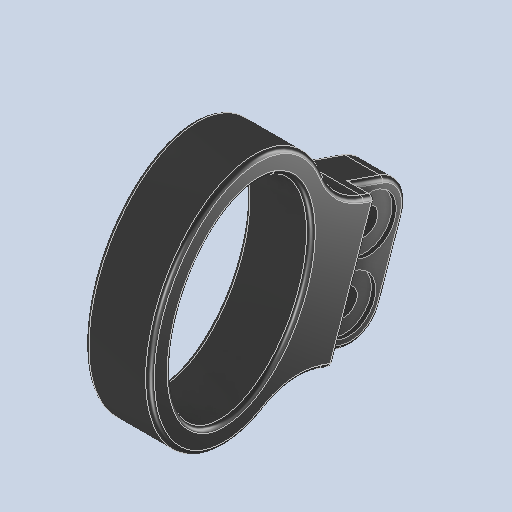
# Autodesk Inventor part: TorsoFrontBumper
Saved by Autodesk Inventor 2024.2 (Build 282272000, 272)
## iProperties
Created: 2024-01-21
Part Number: TorsoFrontBumper
Material: ABS Plastic
Document SubType Name: Modeling
Designer: Masato Kubotera
Density: 1.06 g/cm^3
Appearance: Glossy - Black
Mass: 18.7145 g
Surface Area: 72.9359 cm^2
Volume: 17.6552 cm^3
Catalog Web Link: https://www.poly-maker.jp/polyflex-tpu90.html
Author: Masato Kubotera
Autodesk Inventor part; units mm, degrees
ref_plane "YZ Plane" through (0, 0, 0) normal (1, 0, 0) x (0, 1, 0)
ref_plane "XZ Plane" through (0, 0, 0) normal (0, 1, 0) x (-1, 0, 0)
ref_plane "XY Plane" through (0, 0, 0) normal (0, 0, 1) x (1, 0, 0)
derived "TorsoSideFrame.ipt"
sketch "Sketch5" plane through (0, 0, 0) normal (0, 1, 0) x (-1, 0, 0)
  ellipse E0 centre (-84.0749, 16.6972) end of major axis (-76.7401, 37.9681) minor radius 15 projected
  ellipse E1 centre (-84.0749, 16.6972) end of major axis (-93.0397, -9.3006) minor radius 20 projected
  line L0 (-63.4041, 25.9649) -> (-39.2683, 17.6422) projected
  line L1 (-49.374, -11.6643) -> (-73.5098, -3.3416) projected
  line L2 (-39.2683, 17.6422) -> (-49.374, -11.6643) projected
  line L3 (-48.2759, 36) -> (-65, -12.5) projected
  point P0 (0, 0)
  point P1 (-54.4839, -1.1756)
  point P2 (-49.757, 12.5323)
  point P3 (-63.0819, -6.9375)
  point P4 (-52.9762, 22.3691)
  constraints: 1 other
extrude "Extrusion2" add sketch "Sketch5" against normal blind 10
extrude "Extrusion5" add sketch "Sketch5" along normal blind 5 contours E1 | E1 L0 L3 L1
hole "Hole3" at (54.4839, 0, -1.1756) at (49.757, 0, 12.5323) direction (0, -1, 0) diameter 6 end through all counterbore diameter 12.5 counterbore depth 1
fillet "Fillet9" radius 15 4 edges at (63.4041, -5, 25.9649) (63.4041, 2.5, 25.9649) (73.5098, -5, -3.3416) (73.5098, 2.5, -3.3416)
fillet "Fillet10" radius 1 17 edges at (91.4097, -10, -4.5737) (102.9824, -10, 23.217) (91.4097, 5, -4.5737) (44.3211, -10, 2.989) (57.6584, -10, -8.8076) (47.5527, -10, 20.4989) (52.9762, 2.5, 22.3691) (63.0819, 2.5, -6.9375) (46.1222, 0, 20.0057) (56.2279, 0, -9.3009) (44.3211, 0, 2.989) (54.4066, 5, 22.8624) (102.9824, 5, 23.217) (72.3744, 5, -5.211) (64.5123, 5, -6.4442) (61.3578, 5, 26.7371) (58.029, 5, 7.7158)
fillet "Fillet11" radius 7.5 2 edges at (39.2683, -5, 17.6422) (49.374, -5, -11.6643)
sketch "Sketch1" plane through (0, 0, 0) normal (0, 1, 0) x (-1, 0, 0)
  circle A0 centre (0, 0) radius 18.75 projected
  line L0 (0, 0) -> (0, -161.5) projected
  circle A1 centre (0, 0) radius 29 construction
  line L1 (0, 0) -> (0, 36) projected
  line L2 (0, 36) -> (-48.2759, 36) projected
  line L3 (-65, -12.5) -> (-65, -118) projected
  line L4 (-50, -161.5) -> (-35, -161.5) projected
  line L5 (-35, -161.5) -> (-35, -166.5) projected
  line L6 (-35, -166.5) -> (-10, -166.5) projected
  line L7 (-10, -166.5) -> (-10, -161.5) projected
  line L8 (-10, -161.5) -> (0, -161.5) projected
  line L9 (-60, -40.225) -> (-65, -40.225) projected
  line L10 (-44, -161.5) -> (-44, -155.5) construction
  line L11 (-22.5, -166.5) -> (-22.5, -161.5) construction
  arc A2 (-6, -161.5) -> (-10, -161.5) centre (-8, -161.5) ccw projected
  arc A3 (-35, -161.5) -> (-39, -161.5) centre (-37, -161.5) ccw projected
  line L12 (-65, -12.5) -> (-60, -12.5) construction
  line L13 (-60, -12.5) -> (-60, -106) construction
  line L14 (-62.5, -12.5) -> (-62.5, -106) construction
  line L15 (-65, -40.25) -> (-60, -40.25) construction
  arc A4 (-60, -44.225) -> (-60, -40.225) centre (-60, -42.225) ccw projected
  line L16 (-60, -111) -> (0, -111) construction
  line L17 (-60, -106) -> (0, -106) construction
  line L18 (-60, -108.5) -> (-17.75, -108.5) construction
  line L19 (-9.95, -111.05) -> (-25.55, -111.05) projected
  line L20 (-25.55, -111.05) -> (-25.55, -105.95) projected
  line L21 (-25.55, -105.95) -> (-9.95, -105.95) projected
  line L22 (-9.95, -105.95) -> (-9.95, -111.05) projected
  line L23 (-9.95, -111.05) -> (-25.55, -105.95) construction
  line L24 (-25.55, -111.05) -> (-9.95, -105.95) construction
  line L25 (-25.5, -106) -> (-25.5, -111) construction
  arc A5 (-21.55, -105.95) -> (-25.55, -105.95) centre (-23.55, -105.95) ccw projected
  arc A6 (-25.55, -111.05) -> (-21.55, -111.05) centre (-23.55, -111.05) ccw projected
  line L26 (-22.5, -76.5) -> (-42.5, -76.5) construction
  line L27 (-42.5, -76.5) -> (-42.5, -96.5) construction
  line L28 (-42.5, -96.5) -> (-22.5, -96.5) construction
  line L29 (-22.5, -96.5) -> (-22.5, -76.5) construction
  line L30 (-22.5, -76.5) -> (-42.5, -96.5) construction
  line L31 (-42.5, -76.5) -> (-22.5, -96.5) construction
  line L32 (-45, -74) -> (-20, -74) construction
  line L33 (-20, -74) -> (-20, -99) construction
  line L34 (-20, -99) -> (-45, -99) construction
  line L35 (-45, -99) -> (-45, -74) construction
  line L36 (-45, -74) -> (-20, -99) construction
  line L37 (-20, -74) -> (-45, -99) construction
  line L38 (-50, 31) -> (0, 31) construction
  line L39 (-38.05, 31.05) -> (-13.95, 31.05) projected
  line L40 (-13.95, 31.05) -> (-13.95, 25.95) projected
  line L41 (-13.95, 25.95) -> (-38.05, 25.95) projected
  line L42 (-38.05, 25.95) -> (-38.05, 31.05) projected
  line L43 (-38.05, 31.05) -> (-13.95, 25.95) construction
  line L44 (-13.95, 31.05) -> (-38.05, 25.95) construction
  line L45 (-38.05, 28.5) -> (-13.95, 28.5) construction
  line L46 (-38, 31) -> (-38, 26) construction
  line L47 (-26, 31.05) -> (-26, 25.95) construction
  line L48 (-14, 31) -> (-14, 26) construction
  arc A7 (-34.05, 31.05) -> (-38.05, 31.05) centre (-36.05, 31.05) ccw projected
  arc A8 (-38.05, 25.95) -> (-34.05, 25.95) centre (-36.05, 25.95) ccw projected
  arc A9 (-13.95, 31.05) -> (-17.95, 31.05) centre (-15.95, 31.05) ccw projected
  arc A10 (-17.95, 25.95) -> (-13.95, 25.95) centre (-15.95, 25.95) ccw projected
  line L49 (-46.0671, -156.5) -> (-3.5, -156.5) projected
  arc A11 (-47.9578, -155.152) -> (-46.0671, -156.5) centre (-46.0671, -154.5) ccw projected
  arc A12 (-3.5, -156.5) -> (-1.5, -154.5) centre (-3.5, -154.5) ccw projected
  line L50 (-56, -105.25) -> (-29.4627, -105.25) projected
  circle A13 centre (-41.25, -65.25) radius 2 construction
  line L51 (-1.5, -63.25) -> (-56, -63.25) projected
  line L52 (0, 0) -> (-29, 0) construction
  line L53 (-60, -111.75) -> (-29.4627, -111.75) projected
  arc A14 (-27.6434, -112.9192) -> (-20.2699, -114.1308) centre (-23.55, -111.05) ccw projected
  line L54 (-1.5, -154.5) -> (-1.5, -113.75) projected
  arc A15 (-1.5, -113.75) -> (-3.5, -111.75) centre (-3.5, -113.75) ccw projected
  arc A16 (-27.6434, -112.9192) -> (-29.4627, -111.75) centre (-29.4627, -113.75) ccw projected
  circle A17 centre (-33.5, -108.5) radius 1.75 construction
  arc A18 (-18.8121, -113.5) -> (-20.2699, -114.1308) centre (-18.8121, -115.5) ccw projected
  line L55 (-17.75, -105.95) -> (-17.75, -111.05) construction
  arc A19 (-29.4627, -105.25) -> (-27.6434, -104.0808) centre (-29.4627, -103.25) ccw projected
  arc A20 (-20.2699, -102.8692) -> (-27.6434, -104.0808) centre (-23.55, -105.95) ccw projected
  arc A21 (-20.2699, -102.8692) -> (-18.8121, -103.5) centre (-18.8121, -101.5) ccw projected
  line L56 (-10, -106) -> (-10, -111) construction
  arc A22 (-13.95, -111.05) -> (-9.95, -111.05) centre (-11.95, -111.05) ccw projected
  arc A23 (-6.0373, -111.75) -> (-7.8566, -112.9192) centre (-6.0373, -113.75) ccw projected
  arc A24 (-15.2301, -114.1308) -> (-16.6879, -113.5) centre (-16.6879, -115.5) ccw projected
  arc A25 (-15.2301, -114.1308) -> (-7.8566, -112.9192) centre (-11.95, -111.05) ccw projected
  arc A26 (-9.95, -105.95) -> (-13.95, -105.95) centre (-11.95, -105.95) ccw projected
  arc A27 (-16.6879, -103.5) -> (-15.2301, -102.8692) centre (-16.6879, -101.5) ccw projected
  arc A28 (-7.8566, -104.0808) -> (-15.2301, -102.8692) centre (-11.95, -105.95) ccw projected
  arc A29 (-7.8566, -104.0808) -> (-6.0373, -105.25) centre (-6.0373, -103.25) ccw projected
  line L57 (-18.8121, -103.5) -> (-16.6879, -103.5) projected
  line L58 (-18.8121, -113.5) -> (-16.6879, -113.5) projected
  line L59 (-6.0373, -111.75) -> (-3.5, -111.75) projected
  line L60 (-6.0373, -105.25) -> (-3.5, -105.25) projected
  arc A30 (-3.5, -105.25) -> (-1.5, -103.25) centre (-3.5, -103.25) ccw projected
  line L61 (-41.25, -65.25) -> (-36.25, -65.25) construction
  line L62 (-60, -44.225) -> (-60, -86.275) projected
  line L63 (-60, -65.25) -> (-65, -65.25) construction
  line L64 (-65, -90.25) -> (-60, -90.25) construction
  arc A31 (-60, -90.275) -> (-60, -86.275) centre (-60, -88.275) ccw projected
  line L65 (-60, -90.275) -> (-65, -90.275) projected
  line L66 (-60, -106) -> (-65, -106) construction
  line L67 (-1.5, -22.4499) -> (-1.5, -63.25) projected
  line L68 (-56, -67.75) -> (-1.5, -67.75) projected
  line L69 (-1.5, -67.75) -> (-1.5, -103.25) projected
  line L70 (-56, -63.25) -> (-56, -46.6971) projected
  circle A32 centre (-32.5, -86.5) radius 10 projected
  line L71 (-56, -67.75) -> (-56, -105.25) projected
  circle A33 centre (-32.5, -86.5) radius 11 projected
  arc A34 (-14.0872, 17.5443) -> (-22.2374, 3.4277) centre (0, 0) ccw projected
  arc A35 (-22.2374, -3.4277) -> (-14.0872, -17.5443) centre (0, 0) ccw projected
  arc A36 (-8.1502, -20.972) -> (-1.5, -22.4499) centre (0, 0) ccw projected
  arc A37 (-22.2374, 3.4277) -> (-22.2374, -3.4277) centre (-24.75, 0) ccw projected
  line L72 (-48.2759, 36) -> (-65, -12.5) projected
  arc A38 (-42.9869, 36) -> (-50, 31) centre (-42.9869, 28.5817) ccw projected
  line L73 (-75.1102, 42.6949) -> (-93.0397, -9.3006) construction
  ellipse E0 centre (-84.0749, 16.6972) end of major axis (-76.7401, 37.9681) minor radius 15 construction
  ellipse E1 centre (-84.0749, 16.6972) end of major axis (-93.0397, -9.3006) minor radius 20 construction
  line L74 (-75.1102, 42.6949) -> (-76.7401, 37.9681) construction
  line L75 (-105, 43.5) -> (-105, 11.4504) construction
  line L76 (-84.0749, 16.6972) -> (-58.029, 7.7158) construction
  line L77 (-63.4041, 25.9649) -> (-39.2683, 17.6422) construction
  line L78 (-39.2683, 17.6422) -> (-49.374, -11.6643) construction
  line L79 (-49.374, -11.6643) -> (-73.5098, -3.3416) construction
  line L80 (-79.9787, 43.5) -> (-105, 43.5) construction
  line L81 (-47.0676, 20.3317) -> (-57.1733, -8.9749) construction
  circle A39 centre (-49.757, 12.5323) radius 6.25 construction
  circle A40 centre (-54.4839, -1.1756) radius 6.25 construction
  line L82 (-1, 13.5) -> (-28, 13.5) construction
  line L83 (-28, 13.5) -> (-28, -13.5) construction
  line L84 (-28, -13.5) -> (-1, -13.5) construction
  line L85 (-1, -13.5) -> (-1, 13.5) construction
  line L86 (-1, 13.5) -> (-28, -13.5) construction
  line L87 (-28, 13.5) -> (-1, -13.5) construction
  line L88 (0, -65.25) -> (-65, -65.25) construction
  line L89 (-50, -161.5) -> (-65, -118) projected
  line L90 (-16.326, 23) -> (-48.5275, 23) projected
  arc A41 (-16.326, 23) -> (-14.0872, 17.5443) centre (-12.375, 21.4341) ccw projected
  arc A42 (-56, -46.6971) -> (-60, -36.225) centre (-60, -42.225) ccw projected
  arc A43 (-48.7278, 6.3677) -> (-49.9833, 18.7782) centre (-49.757, 12.5323) ccw projected
  arc A44 (-48.7278, 6.3677) -> (-49.8737, 3.0445) centre (-48.3985, 4.395) ccw projected
  arc A45 (-58.5118, -5.9545) -> (-49.8737, 3.0445) centre (-54.4839, -1.1756) ccw projected
  line L91 (-48.5275, 23) -> (-49.9833, 18.7782) projected
  line L92 (-38, 26) -> (-14, 26) construction
  line L93 (-58.5118, -5.9545) -> (-60, -10.2703) projected
  line L94 (-60, -36.225) -> (-60, -10.2703) projected
  line L95 (-31.2796, -23.3529) -> (-31.2796, -46.6256) construction
  line L96 (-46.2796, -23.3529) -> (-46.2796, -46.6256) construction
  line L97 (-31.2796, -23.3529) -> (-46.2796, -23.3529) construction
  line L98 (-31.2796, -46.6256) -> (-46.2796, -46.6256) construction
  arc A46 (-14.0872, -17.5443) -> (-8.1502, -20.972) centre (-12.375, -21.4341) ccw projected
  line L99 (-47.9578, -155.152) -> (-49.9833, -149.2782) projected
  arc A47 (-49.9833, -149.2782) -> (-48.7278, -136.8677) centre (-49.757, -143.0323) ccw projected
  arc A48 (-49.8737, -133.5445) -> (-48.7278, -136.8677) centre (-48.3985, -134.895) ccw projected
  arc A49 (-49.8737, -133.5445) -> (-58.5118, -124.5455) centre (-54.4839, -129.3244) ccw projected
  line L100 (-58.5118, -124.5455) -> (-60, -120.2297) projected
  line L101 (-60, -120.2297) -> (-60, -111.75) projected
  circle A50 centre (-41.25, -65.25) radius 1 construction
  line L102 (-45, -86.5) -> (-20, -86.5) construction
  point P0 (-16.05, -9.6933)
  point P1 (-12.375, -21.4341)
  point P2 (12.375, -21.4341)
  point P3 (24.75, 0)
  point P4 (12.375, 21.4341)
  point P5 (-26, 28.5)
  point P6 (0, -130.75)
  point P7 (0, -158.0887)
  point P8 (-46, 28.5)
  point P9 (-61.4811, -99)
  point P10 (-1.5, -156.5)
  point P11 (-5, -161.5)
  point P12 (-27.9952, -111.75)
  point P13 (-28.0239, -110.5665)
  point P14 (-7.5048, -111.75)
  point P15 (-38, 28.5)
  point P16 (-14.5, 0)
  point P17 (-1, 0)
  point P18 (0, 22.5)
  point P19 (-62.5, -30.25)
  point P20 (-62.5, -100.25)
  constraints: 5 other
body "Solid2"
